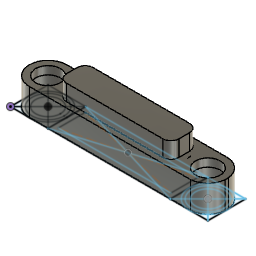
Timer battery adapter (Autodesk Fusion 360 design; units mm, degrees)
Autodesk Fusion 360 part; units mm, degrees
note: some values were not read from the file. Set by a fixed rule: which sketch regions a step uses.
sketch "Sketch1" plane through (0, 0, 0) normal (0, 0, 1) x (1, 0, 0)
  line L0 (0, 0) -> (7, 0)
  line L1 (7, 0) -> (7, 7)
  line L2 (7, 7) -> (0, 7)
  line L3 (0, 7) -> (0, 0)
  line L4 (7, 0) -> (29.8, 0)
  line L5 (29.8, 0) -> (29.8, 7)
  line L6 (29.8, 7) -> (7, 7)
  line L7 (7, 7) -> (7, 0)
  line L8 (29.8, 0) -> (36.8, 0)
  line L9 (36.8, 0) -> (36.8, 7)
  line L10 (36.8, 7) -> (29.8, 7)
  line L11 (29.8, 7) -> (29.8, 0)
  line L12 (0, 7) -> (7, 0)
  line L13 (0, 0) -> (7, 7)
  line L14 (29.8, 7) -> (36.8, 0)
  line L15 (29.8, 0) -> (36.8, 7)
  circle A0 centre (3.5, 3.5) radius 2.3
  circle A1 centre (33.3, 3.5) radius 2.3
  circle A2 centre (3.5, 3.5) radius 3.5
  circle A3 centre (33.3, 3.5) radius 3.5128
  circle A4 centre (33.3, 3.5) radius 3
  circle A5 centre (3.5, 3.5) radius 3
  line L16 (29.8, 7) -> (7, 0)
  line L17 (29.8, 0) -> (7, 7)
  line L18 (7.9, 1) -> (28.9, 1)
  line L19 (28.9, 1) -> (28.9, 6)
  line L20 (28.9, 6) -> (7.9, 6)
  line L21 (7.9, 6) -> (7.9, 1)
  line L22 (7.9, 1) -> (28.9, 6) construction
  line L23 (28.9, 1) -> (7.9, 6) construction
  point P0 (18.4, 3.5)
  dimension "d1" = 7
  dimension "d2" = 7
  dimension "d3" = 22.8
  dimension "d4" = 7
  dimension "d5" = 4.6
  dimension "d6" = 4.6
  dimension "d9" = 6
  dimension "d10" = 6
  dimension "d13" = 21
  dimension "d14" = 5
  constraint horizontal L0
  constraint vertical L1
  constraint horizontal L2
  constraint vertical L3
  constraint coincident L0.start L3.end
  constraint horizontal L4
  constraint vertical L5
  constraint horizontal L6
  constraint vertical L7
  constraint horizontal L8
  constraint vertical L9
  constraint horizontal L10
  constraint vertical L11
  constraint midpoint L13 A0.centre
  constraint midpoint L14 A1.centre
  constraint concentric A0 A2
  constraint tangent L0 A2
  constraint concentric A1 A3
  constraint concentric A3 A4
  constraint concentric A0 A5
  constraint horizontal L18
  constraint perpendicular L18 L19
  constraint parallel L18 L20
  constraint parallel L19 L21
  constraint coincident L22 P0
  constraint coincident L23 P0
  constraint midpoint L17 P0
  measures "d1" distance of L0.start L0.end
  measures "d2" distance of L0.start L2.end
  measures "d3" distance of L0.end L4.end
  measures "d4" distance of L4.end L8.end
  measures "d5" diameter of A0
  measures "d6" diameter of A1
  measures "d9" diameter of A4
  measures "d10" diameter of A5
  measures "d13" distance of L19.end L20.end
  measures "d14" distance of L18.end L19.end
extrude "Extrude1" add sketch "Sketch1" along normal blind 5 contours L0 L12 A2 | L12 L13 A2 A5 | L12 L13 A2 A5 | L1 L7 L12 A2 | L4 L16 L17 L18 | L1 L7 L16 L17 L18 L20 L21 | L12 L13 A2 A5 | L12 L13 A2 A5 | L12 L13 A0 A5 | L12 L13 A0 A5 | L1 L7 L13 A2 | L5 L11 A3 L16 L17 L18 L19 L20 | L8 L15 A3 | L5 L11 L15 A3 | L16 L17 L18 L20 L21 | L16 L17 L18 | L12 L13 A0 A5 | L2 L13 A2 | L12 L13 A0 A5 | L6 L16 L17 L20 | L5 L11 L14 L15 A3 A4 | L8 L14 L15 A3 A4 | L16 L17 L18 L19 L20 | L16 L17 L20 | L5 L11 L14 A3 | L10 L14 A3 | L14 L15 A1 A4 | L14 L15 A1 A4 | L10 L14 L15 A3 A4 | L9 L14 L15 A3 A4 | L14 L15 A1 A4 | L14 L15 A1 A4
extrude "Extrude2" cut sketch "Sketch1" along normal blind 3.5 contours L12 L13 A0 A5 | L12 L13 A0 A5 | L12 L13 A0 A5 | L12 L13 A0 A5 | L14 L15 A1 A4 | L14 L15 A1 A4 | L14 L15 A1 A4 | L14 L15 A1 A4
extrude "Extrude3" add sketch "Sketch1" along normal blind 8 contours L16 L17 L18 L20 L21 | L16 L17 L18 | L16 L17 L18 L19 L20 | L16 L17 L20
fillet "Fillet1" radius 1.5 1 edges at (7.9, 6, 6.5)
fillet "Fillet2" radius 1.5 1 edges at (7.9, 1, 6.5)
fillet "Fillet3" radius 1.5 1 edges at (28.9, 6, 6.5)
fillet "Fillet4" radius 1.5 1 edges at (28.9, 1, 6.5)
